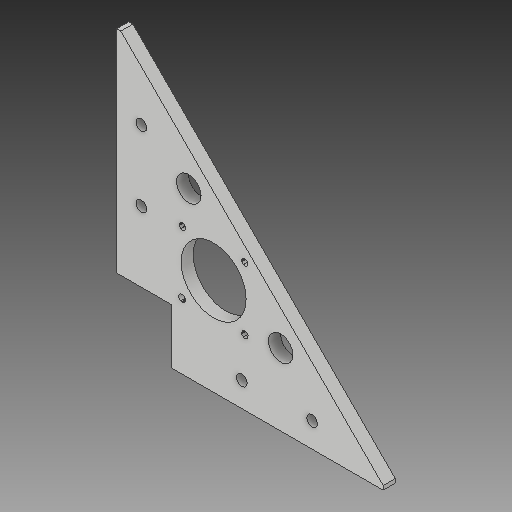
# Autodesk Inventor part: Z Motor Mount Right
Saved by Autodesk Inventor 2018 (Build 220112000, 112)
## iProperties
Created: 2016-07-25
Part Number: Z Motor Mount Right
Material: Generic
Document SubType Name: Modeling
Designer: User
Density: 1 g/cm^3
Appearance: Default
Author: User
Autodesk Inventor part; units mm, degrees
ref_plane "YZ Plane" through (0, 0, 0) normal (1, 0, 0) x (0, 1, 0)
ref_plane "XZ Plane" through (0, 0, 0) normal (0, 1, 0) x (-1, 0, 0)
ref_plane "XY Plane" through (0, 0, 0) normal (0, 0, 1) x (1, 0, 0)
sketch "Sketch1" plane through (0, 0, 0) normal (0, 0, 1) x (1, 0, 0)
  line L0 (141.1314, 655.2458) -> (140.8814, 655.8708)
  line L1 (140.8814, 655.8708) -> (140.4815, 656.3958)
  line L2 (140.4815, 656.3958) -> (139.9565, 656.7958)
  line L3 (139.9565, 656.7958) -> (139.3565, 657.0458)
  line L4 (139.3565, 657.0458) -> (138.7065, 657.1208)
  line L5 (138.7065, 657.1208) -> (138.0565, 657.0457)
  line L6 (138.0565, 657.0457) -> (137.4315, 656.7958)
  line L7 (137.4315, 656.7958) -> (136.9065, 656.3958)
  line L8 (136.9065, 656.3958) -> (136.5065, 655.8708)
  line L9 (136.5065, 655.8708) -> (136.2565, 655.2458)
  line L10 (136.2565, 655.2458) -> (136.1815, 654.5958)
  line L11 (136.1815, 654.5958) -> (136.2565, 653.9458)
  line L12 (136.2565, 653.9458) -> (136.5066, 653.3458)
  line L13 (136.5066, 653.3458) -> (136.9065, 652.8208)
  line L14 (136.9065, 652.8208) -> (137.4315, 652.4208)
  line L15 (137.4315, 652.4208) -> (138.0566, 652.1708)
  line L16 (138.0566, 652.1708) -> (138.7065, 652.0958)
  line L17 (138.7065, 652.0958) -> (139.3565, 652.1708)
  line L18 (139.3565, 652.1708) -> (139.9565, 652.4209)
  line L19 (139.9565, 652.4209) -> (140.4815, 652.8208)
  line L20 (140.4815, 652.8208) -> (140.8815, 653.3458)
  line L21 (140.8815, 653.3458) -> (141.1316, 653.9458)
  line L22 (141.1316, 653.9458) -> (141.2315, 654.5952)
  line L23 (141.2315, 654.5952) -> (141.1314, 655.2458)
  line L24 (141.1315, 620.3958) -> (140.8816, 621.0208)
  line L25 (140.8816, 621.0208) -> (140.4817, 621.5458)
  line L26 (140.4817, 621.5458) -> (139.9567, 621.9458)
  line L27 (139.9567, 621.9458) -> (139.3567, 622.1958)
  line L28 (139.3567, 622.1958) -> (138.7067, 622.2708)
  line L29 (138.7067, 622.2708) -> (138.0565, 622.1957)
  line L30 (138.0565, 622.1957) -> (137.4315, 621.9458)
  line L31 (137.4315, 621.9458) -> (136.9065, 621.5458)
  line L32 (136.9065, 621.5458) -> (136.5065, 621.0208)
  line L33 (136.5065, 621.0208) -> (136.2565, 620.3958)
  line L34 (136.2565, 620.3958) -> (136.1815, 619.7458)
  line L35 (136.1815, 619.7458) -> (136.2565, 619.0958)
  line L36 (136.2565, 619.0958) -> (136.5066, 618.4958)
  line L37 (136.5066, 618.4958) -> (136.9065, 617.9708)
  line L38 (136.9065, 617.9708) -> (137.4315, 617.5708)
  line L39 (137.4315, 617.5708) -> (138.0566, 617.3208)
  line L40 (138.0566, 617.3208) -> (138.7065, 617.2208)
  line L41 (138.7065, 617.2208) -> (139.3565, 617.3208)
  line L42 (139.3565, 617.3208) -> (139.9565, 617.5708)
  line L43 (139.9565, 617.5708) -> (140.4815, 617.9708)
  line L44 (140.4815, 617.9708) -> (140.8815, 618.4957)
  line L45 (140.8815, 618.4957) -> (141.1315, 619.0958)
  line L46 (141.1315, 619.0958) -> (141.2316, 619.7458)
  line L47 (141.2316, 619.7458) -> (141.1315, 620.3958)
  line L48 (160.5564, 621.6955) -> (160.4065, 622.0705)
  line L49 (160.4065, 622.0705) -> (160.1565, 622.3956)
  line L50 (160.1565, 622.3956) -> (159.8315, 622.6456)
  line L51 (159.8315, 622.6456) -> (159.4315, 622.8206)
  line L52 (159.4315, 622.8206) -> (159.0316, 622.8707)
  line L53 (159.0316, 622.8707) -> (158.6065, 622.8207)
  line L54 (158.6065, 622.8207) -> (158.2315, 622.6458)
  line L55 (158.2315, 622.6458) -> (157.9065, 622.3958)
  line L56 (157.9065, 622.3958) -> (157.6565, 622.0708)
  line L57 (157.6565, 622.0708) -> (157.4815, 621.6958)
  line L58 (157.4815, 621.6958) -> (157.4315, 621.2708)
  line L59 (157.4315, 621.2708) -> (157.4815, 620.8708)
  line L60 (157.4815, 620.8708) -> (157.6565, 620.4958)
  line L61 (157.6565, 620.4958) -> (157.9065, 620.1458)
  line L62 (157.9065, 620.1458) -> (158.2315, 619.8957)
  line L63 (158.2315, 619.8957) -> (158.6065, 619.7457)
  line L64 (158.6065, 619.7457) -> (159.0315, 619.6957)
  line L65 (159.0315, 619.6957) -> (159.4314, 619.7457)
  line L66 (159.4314, 619.7457) -> (159.8315, 619.8957)
  line L67 (159.8315, 619.8957) -> (160.1565, 620.1457)
  line L68 (160.1565, 620.1457) -> (160.4063, 620.4956)
  line L69 (160.4063, 620.4956) -> (160.5563, 620.8706)
  line L70 (160.5563, 620.8706) -> (160.6063, 621.2705)
  line L71 (160.6063, 621.2705) -> (160.5564, 621.6955)
  line L72 (189.9814, 609.9208) -> (188.3815, 613.7708)
  line L73 (188.3815, 613.7708) -> (185.8314, 617.0958)
  line L74 (185.8314, 617.0958) -> (182.5315, 619.6458)
  line L75 (182.5315, 619.6458) -> (178.6565, 621.2458)
  line L76 (178.6565, 621.2458) -> (174.5315, 621.7708)
  line L77 (174.5315, 621.7708) -> (170.3815, 621.2458)
  line L78 (170.3815, 621.2458) -> (166.5315, 619.6458)
  line L79 (166.5315, 619.6458) -> (163.2065, 617.0958)
  line L80 (163.2065, 617.0958) -> (160.6815, 613.7708)
  line L81 (160.6815, 613.7708) -> (159.0815, 609.9208)
  line L82 (159.0815, 609.9208) -> (158.5315, 605.7708)
  line L83 (158.5315, 605.7708) -> (159.0815, 601.6458)
  line L84 (159.0815, 601.6458) -> (160.6815, 597.7708)
  line L85 (160.6815, 597.7708) -> (163.2065, 594.4708)
  line L86 (163.2065, 594.4708) -> (166.5315, 591.9208)
  line L87 (166.5315, 591.9208) -> (170.3815, 590.3207)
  line L88 (170.3815, 590.3207) -> (174.5315, 589.7708)
  line L89 (174.5315, 589.7708) -> (178.6565, 590.3207)
  line L90 (178.6565, 590.3207) -> (182.5314, 591.9208)
  line L91 (182.5314, 591.9208) -> (185.8314, 594.4708)
  line L92 (185.8314, 594.4708) -> (188.3814, 597.7708)
  line L93 (188.3814, 597.7708) -> (189.9815, 601.6458)
  line L94 (189.9815, 601.6458) -> (190.5315, 605.7706)
  line L95 (190.5315, 605.7706) -> (189.9814, 609.9208)
  line L96 (191.5564, 621.6955) -> (191.4065, 622.0705)
  line L97 (191.4065, 622.0705) -> (191.1565, 622.3955)
  line L98 (191.1565, 622.3955) -> (190.8315, 622.6456)
  line L99 (190.8315, 622.6456) -> (190.4315, 622.8206)
  line L100 (190.4315, 622.8206) -> (190.0316, 622.8706)
  line L101 (190.0316, 622.8706) -> (189.6064, 622.8207)
  line L102 (189.6064, 622.8207) -> (189.2315, 622.6458)
  line L103 (189.2315, 622.6458) -> (188.9065, 622.3958)
  line L104 (188.9065, 622.3958) -> (188.6565, 622.0708)
  line L105 (188.6565, 622.0708) -> (188.4815, 621.6958)
  line L106 (188.4815, 621.6958) -> (188.4315, 621.2708)
  line L107 (188.4315, 621.2708) -> (188.4815, 620.8708)
  line L108 (188.4815, 620.8708) -> (188.6565, 620.4958)
  line L109 (188.6565, 620.4958) -> (188.9065, 620.1458)
  line L110 (188.9065, 620.1458) -> (189.2315, 619.8957)
  line L111 (189.2315, 619.8957) -> (189.6064, 619.7457)
  line L112 (189.6064, 619.7457) -> (190.0315, 619.6957)
  line L113 (190.0315, 619.6957) -> (190.4314, 619.7457)
  line L114 (190.4314, 619.7457) -> (190.8314, 619.8957)
  line L115 (190.8314, 619.8957) -> (191.1565, 620.1457)
  line L116 (191.1565, 620.1457) -> (191.4063, 620.4956)
  line L117 (191.4063, 620.4956) -> (191.5563, 620.8706)
  line L118 (191.5563, 620.8706) -> (191.6063, 621.2707)
  line L119 (191.6063, 621.2707) -> (191.5564, 621.6955)
  line L120 (213.5818, 594.921) -> (212.9818, 596.371)
  line L121 (212.9818, 596.371) -> (212.0318, 597.596)
  line L122 (212.0318, 597.596) -> (210.7817, 598.5708)
  line L123 (210.7817, 598.5708) -> (209.3317, 599.1709)
  line L124 (209.3317, 599.1709) -> (207.7817, 599.3708)
  line L125 (207.7817, 599.3708) -> (206.2317, 599.1709)
  line L126 (206.2317, 599.1709) -> (204.7817, 598.5708)
  line L127 (204.7817, 598.5708) -> (203.5317, 597.5958)
  line L128 (203.5317, 597.5958) -> (202.5817, 596.3708)
  line L129 (202.5817, 596.3708) -> (201.9817, 594.9208)
  line L130 (201.9817, 594.9208) -> (201.7817, 593.3708)
  line L131 (201.7817, 593.3708) -> (201.9817, 591.8208)
  line L132 (201.9817, 591.8208) -> (202.5818, 590.3708)
  line L133 (202.5818, 590.3708) -> (203.5318, 589.1209)
  line L134 (203.5318, 589.1209) -> (204.7819, 588.1709)
  line L135 (204.7819, 588.1709) -> (206.2319, 587.5709)
  line L136 (206.2319, 587.5709) -> (207.7819, 587.3709)
  line L137 (207.7819, 587.3709) -> (209.3319, 587.5709)
  line L138 (209.3319, 587.5709) -> (210.7819, 588.171)
  line L139 (210.7819, 588.171) -> (212.0317, 589.121)
  line L140 (212.0317, 589.121) -> (212.9818, 590.3712)
  line L141 (212.9818, 590.3712) -> (213.5818, 591.8212)
  line L142 (213.5818, 591.8212) -> (213.7818, 593.3712)
  line L143 (213.7818, 593.3712) -> (213.5818, 594.921)
  line L144 (191.5564, 590.6955) -> (191.4065, 591.0705)
  line L145 (191.4065, 591.0705) -> (191.1565, 591.3955)
  line L146 (191.1565, 591.3955) -> (190.8315, 591.6456)
  line L147 (190.8315, 591.6456) -> (190.4315, 591.8206)
  line L148 (190.4315, 591.8206) -> (190.0316, 591.8706)
  line L149 (190.0316, 591.8706) -> (189.6065, 591.8207)
  line L150 (189.6065, 591.8207) -> (189.2315, 591.6458)
  line L151 (189.2315, 591.6458) -> (188.9065, 591.3958)
  line L152 (188.9065, 591.3958) -> (188.6565, 591.0708)
  line L153 (188.6565, 591.0708) -> (188.4815, 590.6958)
  line L154 (188.4815, 590.6958) -> (188.4315, 590.2708)
  line L155 (188.4315, 590.2708) -> (188.4815, 589.8708)
  line L156 (188.4815, 589.8708) -> (188.6565, 589.4958)
  line L157 (188.6565, 589.4958) -> (188.9065, 589.1458)
  line L158 (188.9065, 589.1458) -> (189.2315, 588.8957)
  line L159 (189.2315, 588.8957) -> (189.6064, 588.7457)
  line L160 (189.6064, 588.7457) -> (190.0315, 588.6957)
  line L161 (190.0315, 588.6957) -> (190.4314, 588.7457)
  line L162 (190.4314, 588.7457) -> (190.8314, 588.8957)
  line L163 (190.8314, 588.8957) -> (191.1564, 589.1457)
  line L164 (191.1564, 589.1457) -> (191.4063, 589.4956)
  line L165 (191.4063, 589.4956) -> (191.5563, 589.8706)
  line L166 (191.5563, 589.8706) -> (191.6063, 590.2706)
  line L167 (191.6063, 590.2706) -> (191.5564, 590.6955)
  line L168 (190.9314, 570.5957) -> (190.6815, 571.2208)
  line L169 (190.6815, 571.2208) -> (190.2815, 571.7458)
  line L170 (190.2815, 571.7458) -> (189.7565, 572.1457)
  line L171 (189.7565, 572.1457) -> (189.1566, 572.3958)
  line L172 (189.1566, 572.3958) -> (188.5065, 572.4708)
  line L173 (188.5065, 572.4708) -> (187.8565, 572.3957)
  line L174 (187.8565, 572.3957) -> (187.2315, 572.1458)
  line L175 (187.2315, 572.1458) -> (186.7065, 571.7458)
  line L176 (186.7065, 571.7458) -> (186.3065, 571.2208)
  line L177 (186.3065, 571.2208) -> (186.0565, 570.5958)
  line L178 (186.0565, 570.5958) -> (185.9815, 569.9458)
  line L179 (185.9815, 569.9458) -> (186.0566, 569.2958)
  line L180 (186.0566, 569.2958) -> (186.3066, 568.6958)
  line L181 (186.3066, 568.6958) -> (186.7066, 568.1708)
  line L182 (186.7066, 568.1708) -> (187.2316, 567.7708)
  line L183 (187.2316, 567.7708) -> (187.8566, 567.5208)
  line L184 (187.8566, 567.5208) -> (188.5065, 567.4208)
  line L185 (188.5065, 567.4208) -> (189.1566, 567.5208)
  line L186 (189.1566, 567.5208) -> (189.7565, 567.7708)
  line L187 (189.7565, 567.7708) -> (190.2816, 568.1708)
  line L188 (190.2816, 568.1708) -> (190.6816, 568.6958)
  line L189 (190.6816, 568.6958) -> (190.9316, 569.2958)
  line L190 (190.9316, 569.2958) -> (191.0315, 569.9452)
  line L191 (191.0315, 569.9452) -> (190.9314, 570.5957)
  line L192 (225.7813, 570.5958) -> (225.5313, 571.2209)
  line L193 (225.5313, 571.2209) -> (225.1314, 571.7459)
  line L194 (225.1314, 571.7459) -> (224.6064, 572.1458)
  line L195 (224.6064, 572.1458) -> (224.0064, 572.3958)
  line L196 (224.0064, 572.3958) -> (223.3564, 572.4709)
  line L197 (223.3564, 572.4709) -> (222.7064, 572.3958)
  line L198 (222.7064, 572.3958) -> (222.0814, 572.1458)
  line L199 (222.0814, 572.1458) -> (221.5814, 571.7458)
  line L200 (221.5814, 571.7458) -> (221.1814, 571.2208)
  line L201 (221.1814, 571.2208) -> (220.9064, 570.5958)
  line L202 (220.9064, 570.5958) -> (220.8314, 569.9458)
  line L203 (220.8314, 569.9458) -> (220.9064, 569.2963)
  line L204 (220.9064, 569.2963) -> (221.1814, 568.696)
  line L205 (221.1814, 568.696) -> (221.5813, 568.171)
  line L206 (221.5813, 568.171) -> (222.0814, 567.771)
  line L207 (222.0814, 567.771) -> (222.7063, 567.521)
  line L208 (222.7063, 567.521) -> (223.3563, 567.421)
  line L209 (223.3563, 567.421) -> (224.0063, 567.521)
  line L210 (224.0063, 567.521) -> (224.6063, 567.771)
  line L211 (224.6063, 567.771) -> (225.1313, 568.171)
  line L212 (225.1313, 568.171) -> (225.5313, 568.696)
  line L213 (225.5313, 568.696) -> (225.7813, 569.296)
  line L214 (225.7813, 569.296) -> (225.8813, 569.9456)
  line L215 (225.8813, 569.9456) -> (225.7813, 570.5958)
  line L216 (160.5634, 590.697) -> (160.4134, 591.072)
  line L217 (160.4134, 591.072) -> (160.1634, 591.397)
  line L218 (160.1634, 591.397) -> (159.8134, 591.6469)
  line L219 (159.8134, 591.6469) -> (159.4383, 591.8219)
  line L220 (159.4383, 591.8219) -> (159.0384, 591.8719)
  line L221 (159.0384, 591.8719) -> (158.6133, 591.822)
  line L222 (158.6133, 591.822) -> (158.2383, 591.647)
  line L223 (158.2383, 591.647) -> (157.9133, 591.397)
  line L224 (157.9133, 591.397) -> (157.6633, 591.0721)
  line L225 (157.6633, 591.0721) -> (157.5133, 590.6971)
  line L226 (157.5133, 590.6971) -> (157.4383, 590.2721)
  line L227 (157.4383, 590.2721) -> (157.5133, 589.8721)
  line L228 (157.5133, 589.8721) -> (157.6632, 589.4971)
  line L229 (157.6632, 589.4971) -> (157.9132, 589.1721)
  line L230 (157.9132, 589.1721) -> (158.2381, 588.897)
  line L231 (158.2381, 588.897) -> (158.6131, 588.747)
  line L232 (158.6131, 588.747) -> (159.0381, 588.6969)
  line L233 (159.0381, 588.6969) -> (159.4381, 588.747)
  line L234 (159.4381, 588.747) -> (159.8131, 588.8969)
  line L235 (159.8131, 588.8969) -> (160.1631, 589.172)
  line L236 (160.1631, 589.172) -> (160.4132, 589.4969)
  line L237 (160.4132, 589.4969) -> (160.5632, 589.8719)
  line L238 (160.5632, 589.8719) -> (160.6132, 590.2722)
  line L239 (160.6132, 590.2722) -> (160.5634, 590.697)
  line L240 (128.495, 689.7962) -> (126.495, 689.7958)
  line L241 (126.495, 689.7958) -> (126.518, 584.9458)
  line L242 (126.518, 584.9458) -> (153.718, 584.9517)
  line L243 (153.718, 584.9517) -> (153.7239, 557.7518)
  line L244 (153.7239, 557.7518) -> (258.5739, 557.7747)
  line L245 (258.5739, 557.7747) -> (258.5735, 559.7747)
  line L246 (258.5735, 559.7747) -> (128.495, 689.7962)
  line L247 (168.0123, 640.5721) -> (167.4122, 642.0222)
  line L248 (167.4122, 642.0222) -> (166.4372, 643.2721)
  line L249 (166.4372, 643.2721) -> (165.2123, 644.2221)
  line L250 (165.2123, 644.2221) -> (163.7623, 644.8221)
  line L251 (163.7623, 644.8221) -> (162.2123, 645.0221)
  line L252 (162.2123, 645.0221) -> (160.6623, 644.8221)
  line L253 (160.6623, 644.8221) -> (159.2123, 644.2221)
  line L254 (159.2123, 644.2221) -> (157.9623, 643.272)
  line L255 (157.9623, 643.272) -> (157.0124, 642.022)
  line L256 (157.0124, 642.022) -> (156.4124, 640.572)
  line L257 (156.4124, 640.572) -> (156.2124, 639.022)
  line L258 (156.2124, 639.022) -> (156.4124, 637.472)
  line L259 (156.4124, 637.472) -> (157.0124, 636.022)
  line L260 (157.0124, 636.022) -> (157.9625, 634.7721)
  line L261 (157.9625, 634.7721) -> (159.2125, 633.8221)
  line L262 (159.2125, 633.8221) -> (160.6626, 633.2221)
  line L263 (160.6626, 633.2221) -> (162.2125, 633.0221)
  line L264 (162.2125, 633.0221) -> (163.7626, 633.2221)
  line L265 (163.7626, 633.2221) -> (165.2125, 633.8221)
  line L266 (165.2125, 633.8221) -> (166.4375, 634.7721)
  line L267 (166.4375, 634.7721) -> (167.4122, 636.022)
  line L268 (167.4122, 636.022) -> (168.0123, 637.4721)
  line L269 (168.0123, 637.4721) -> (168.2123, 639.0222)
  line L270 (168.2123, 639.0222) -> (168.0123, 640.5721)
  line L271 (258.4596, 560.9292) -> (260.4596, 560.9297)
  point P0 (0, 0)
  constraints: 544 end point, 13 parallel, 9 perpendicular
extrude "Extrusion1" add sketch "Sketch1" along normal blind 6
sketch "Sketch2" plane through (0, 0, 6) normal (0, 0, 1) x (1, 0, 0)
  line L0 (138.7065, 652.0958) -> (138.0566, 652.1708) projected
  line L1 (138.7065, 657.1436) -> (138.7065, 652.0958)
  line L2 (163.7623, 644.8221) -> (162.2123, 645.0221) projected
  line L3 (162.2125, 633.0221) -> (163.7626, 633.2221) projected
  line L4 (162.2123, 645.0221) -> (162.2125, 633.0221)
  line L5 (189.6064, 622.8207) -> (190.0316, 622.8706) projected
  line L6 (190.4314, 619.7457) -> (190.0315, 619.6957) projected
  line L7 (190.0316, 622.8706) -> (190.0315, 619.6957)
  line L8 (206.2317, 599.1709) -> (207.7817, 599.3708) projected
  line L9 (209.3319, 587.5709) -> (207.7819, 587.3709) projected
  line L10 (207.7817, 599.3708) -> (207.7819, 587.3709)
  line L11 (223.3564, 572.4709) -> (224.0064, 572.3958) projected
  line L12 (224.0063, 567.521) -> (223.3563, 567.421) projected
  line L13 (223.3564, 572.4709) -> (223.3563, 567.421)
  line L14 (188.5065, 572.4708) -> (188.5065, 567.4208)
  line L15 (190.0316, 591.8706) -> (189.6065, 591.8207) projected
  line L16 (189.6064, 588.7457) -> (190.0315, 588.6957) projected
  line L17 (190.0316, 591.8706) -> (190.0315, 588.6957)
  line L18 (158.6133, 591.822) -> (159.0384, 591.8719) projected
  line L19 (159.0381, 588.6969) -> (158.6131, 588.747) projected
  line L20 (159.0384, 591.8719) -> (159.0381, 588.6969)
  line L21 (138.7067, 622.2708) -> (139.3567, 622.1958) projected
  line L22 (139.3565, 617.3208) -> (138.7065, 617.2208) projected
  line L23 (138.7067, 622.2708) -> (138.7065, 617.2208)
  line L24 (159.0316, 622.8707) -> (158.6065, 622.8207) projected
  line L25 (158.6065, 619.7457) -> (159.0315, 619.6957) projected
  line L26 (159.0316, 622.8707) -> (159.0315, 619.6957)
  line L27 (174.5315, 621.7708) -> (178.6565, 621.2458) projected
  line L28 (170.3815, 590.3207) -> (174.5315, 589.7708) projected
  line L29 (174.5315, 621.7708) -> (174.5315, 589.7708)
  circle A0 centre (138.7065, 654.6197) radius 2.65
  circle A1 centre (138.7066, 619.7458) radius 2.65
  circle A2 centre (188.5065, 569.9458) radius 2.65
  circle A3 centre (223.3563, 569.9459) radius 2.65
  circle A4 centre (190.0315, 590.2832) radius 1.6
  circle A5 centre (158.8084, 590.4059) radius 1.6
  circle A6 centre (159.0315, 621.2832) radius 1.6
  circle A7 centre (190.0315, 621.2832) radius 1.6
  circle A8 centre (207.7818, 593.3709) radius 6.1
  circle A9 centre (162.2124, 639.0221) radius 6.1
  circle A10 centre (174.5315, 605.7708) radius 16.1
  point P0 (0, 0)
  dimension "d2" = 5.3
  dimension "d3" = 5.3
  dimension "d4" = 5.3
  dimension "d5" = 5.3
  dimension "d6" = 3.2
  dimension "d7" = 3.2
  dimension "d8" = 3.2
  dimension "d9" = 3.2
  dimension "d10" = 12.2
  dimension "d11" = 12.2
  dimension "d12" = 32.2
  constraints: 22 end point, 11 centre point, 10 midpoint, 1 vertical
  measures "d2" diameter of A0
  measures "d3" diameter of A1
  measures "d4" diameter of A2
  measures "d5" diameter of A3
  measures "d6" diameter of A4
  measures "d7" diameter of A5
  measures "d8" diameter of A6
  measures "d9" diameter of A7
  measures "d10" diameter of A8
  measures "d11" diameter of A9
  measures "d12" diameter of A10
extrude "Extrusion3" cut sketch "Sketch2" against normal blind 6
body "Solid1"
